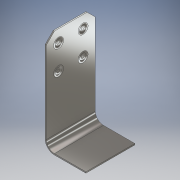
# Autodesk Inventor part: EPS_BatteryTab
Saved by Autodesk Inventor 2018 (Build 220112000, 112)
## iProperties
Created: 2018-06-04
Part Number: EPS_BatteryTab
Material: Nickel-Copper Alloy 400
Document SubType Name: Modeling
Designer: Bradley
Density: 8.83 g/cm^3
Appearance: Chrome - Polished
Author: Bradley
Autodesk Inventor part; units mm, degrees
ref_plane "YZ Plane" through (0, 0, 0) normal (1, 0, 0) x (0, 1, 0)
ref_plane "XZ Plane" through (0, 0, 0) normal (0, 1, 0) x (-1, 0, 0)
ref_plane "XY Plane" through (0, 0, 0) normal (0, 0, 1) x (1, 0, 0)
sketch "Sketch1" plane through (0, 0, 0) normal (0, 1, 0) x (-1, 0, 0)
  line L0 (2.5, 6.075) -> (2.35, 6.075)
  line L1 (2.35, 6.075) -> (2.35, -4.925)
  arc A0 (1.35, -5.925) -> (2.35, -4.925) centre (1.35, -4.925) ccw
  line L2 (1.35, -5.925) -> (-2.5, -5.925)
  line L3 (-2.5, -5.925) -> (-2.5, -6.075)
  line L4 (-2.5, -6.075) -> (1.35, -6.075)
  arc A1 (1.35, -6.075) -> (2.5, -4.925) centre (1.35, -4.925) ccw
  line L5 (2.5, -4.925) -> (2.5, 6.075)
  line L6 (-2.5, -6.075) -> (2.5, -6.075) construction
  line L7 (2.5, -6.075) -> (2.5, 6.075) construction
  point P0 (0, 0)
  point P1 (0, 0)
  point P2 (0, -6.075)
  point P3 (2.5, 0)
  dimension "d0" = 0.15
  dimension "d1" = 12.15
  dimension "d2" = 1
  dimension "d3" = 5
  constraints: 16 end point, 6 perpendicular, 4 point on circle, 3 tangent, 2 centre point, 2 horizontal alignment, 2 midpoint, 2 vertical alignment, 1 concentric, 1 horizontal, 1 parallel, 1 point on line
  measures "d0" distance of L0.start L0.end
  measures "d1" distance between parallel lines of L4 L0
  measures "d2" radius of A0
  measures "d3" distance of L3.end L6.end
extrude "Extrusion1" add sketch "Sketch1" along normal mid plane 6
sketch "Sketch2" plane through (-2.35, -3, -4.925) normal (1, 0, 0) x (0, 0, -1)
  line L0 (0, 0) -> (0, 6) projected
  line L1 (-11, 6) -> (0, 6) projected
  line L2 (-11, 0) -> (-11, 6) projected
  line L3 (0, 0) -> (-11, 0) projected
  line L4 (-6.5, 1.5) -> (-9.5, 1.5) construction
  line L5 (-9.5, 1.5) -> (-9.5, 4.5) construction
  line L6 (-9.5, 4.5) -> (-6.5, 4.5) construction
  line L7 (-6.5, 4.5) -> (-6.5, 1.5) construction
  line L8 (-6.5, 1.5) -> (-9.5, 4.5) construction
  line L9 (-9.5, 1.5) -> (-6.5, 4.5) construction
  line L10 (1.15, 0) -> (1.15, 6) construction
  point P0 (-4.925, 3)
  point P1 (-8, 3)
  point P2 (-8, 3)
  dimension "d6" = 9.15
  dimension "d7" = 3
  constraints: 12 end point, 4 coincident, 3 midpoint, 2 parallel, 2 perpendicular, 1 horizontal, 1 horizontal alignment
  measures "d6" distance from line of point (-8, 3) L10
  measures "d7" distance of L4.end L5.end
hole "Hole1" at (-2.35, -1.5, 4.575) at (-2.35, 1.5, 4.575) at (-2.35, 1.5, 1.575) at (-2.35, -1.5, 1.575) direction (-1, 0, 0) diameter 0.6 depth 0.05
fillet "Fillet1" radius 1 8 edges at (-2.35, -1.5, 4.875) (-2.4, -1.5, 4.875) (-2.35, 1.5, 4.875) (-2.4, 1.5, 4.875) (-2.35, 1.5, 1.875) (-2.4, 1.5, 1.875) (-2.35, -1.5, 1.875) (-2.4, -1.5, 1.875)
chamfer "Chamfer1" distance 1 angle 45 2 edges at (-2.425, -3, 6.075) (-2.425, 3, 6.075)
body "Solid1"
